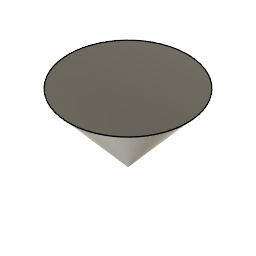
chamfer (Autodesk Fusion 360 design; units mm, degrees)
Autodesk Fusion 360 part; units mm, degrees
sketch "Sketch6" plane through (0, 0, 0) normal (0, 1, 0) x (1, 0, 0)
  line L0 (0, 5.8057) -> (0, -128.793)
  line L1 (0, 5.8057) -> (7.8068, -3.175)
  line L2 (7.8068, -3.175) -> (0, -3.175)
  line L3 (0, 0) -> (5.0468, 0) construction
  line L4 (4.826, 0.254) -> (0, 0.254) construction
  line L5 (1.75, 0) -> (22.5, 0) construction
  dimension "d57" = 41
  dimension "d59" = 0.254
  dimension "d60" = 9.652
  dimension "d61" = 3.175
  constraint vertical L0
  constraint coincident L0 L2.end
  constraint perpendicular L0 L2
  constraint coincident L3.start L0
  constraint coincident L3.start origin
  constraint coincident L1 L3.end
  constraint perpendicular L0 L3
  constraint coincident L0 L4.end
  constraint perpendicular L0 L4
  constraint coincident L1 L4.start
  measures "d57" angle of L0 L1
  measures "d59" distance of L3 L4
  measures "d61" distance of L2 L5
revolve "Revolve1" add sketch "Sketch6" angle 360 about axis through (0, 0, -5.8057) along (0, 0, 1)
equation "d57 = ( 82 / 2 ) * 1 °"
equation "d59 = 0.01 \""
equation "d60 = 0.38 \""
equation "d61 = 0.125 \""
equation "d62 = 0.00 \""
equation "d63 = 0.00 \""
equation "d64 = 0.00 \""
